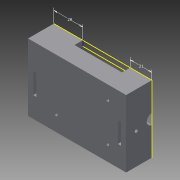
# Autodesk Inventor part: MAINCHAMBER
Saved by Autodesk Inventor 2013 (Build 170138000, 138)
## iProperties
Created: 2013-06-23
Part Number: MAINCHAMBER
Material: Generic
Document SubType Name: Modeling
Designer: Virtual
Density: 1 g/cm^3
Author: Virtual
Autodesk Inventor part; units mm, degrees
ref_plane "YZ Plane" through (0, 0, 0) normal (1, 0, 0) x (0, 1, 0)
ref_plane "XZ Plane" through (0, 0, 0) normal (0, 1, 0) x (-1, 0, 0)
ref_plane "XY Plane" through (0, 0, 0) normal (0, 0, 1) x (1, 0, 0)
sketch "Sketch1" plane through (0, 0, 0) normal (0, 1, 0) x (-1, 0, 0)
  line L0 (0, 0) -> (95, 0)
  line L1 (95, 0) -> (95, 65)
  line L2 (95, 65) -> (0, 65)
  line L3 (0, 65) -> (0, 0)
  dimension "d0" = 95
  dimension "d1" = 65
  constraints: 8 end point, 2 parallel, 1 horizontal, 1 perpendicular
  measures "d0" distance of L2.end L1.end
  measures "d1" distance of L1.end L0.end
extrude "Extrusion1" add sketch "Sketch1" along normal blind 25
sketch "Sketch2" plane through (0, 25, 0) normal (0, 1, 0) x (1, 0, 0)
  line L0 (-5, -5) -> (-90, -5)
  line L1 (-90, -5) -> (-90, -60)
  line L2 (-90, -60) -> (-5, -60)
  line L3 (-5, -60) -> (-5, -5)
  constraints: 8 end point, 2 parallel, 1 horizontal, 1 perpendicular
extrude "Extrusion2" cut sketch "Sketch2" against normal blind 20
sketch "Sketch3" plane through (0, 25, 0) normal (0, 1, 0) x (1, 0, 0)
  line L0 (-5, -60) -> (-90, -60) projected
  line L1 (-95, -65) -> (0, -65) projected
  line L2 (-67, -65) -> (-67, -60)
  line L3 (-21, -60) -> (-21, -65)
  line L4 (-90, -5) -> (-5, -5) projected
  line L5 (0, 0) -> (-95, 0) projected
  line L6 (0, -65) -> (0, 0) projected
  line L7 (-67, -5) -> (-67, 0)
  line L8 (-21, -5) -> (-21, 0)
  line L9 (-67, 0) -> (-21, 0)
  line L10 (-21, -5) -> (-67, -5)
  dimension "d6" = 28
  dimension "d7" = 21
  constraints: 12 end point, 8 point on line, 3 perpendicular, 2 parallel, 1 collinear
  measures "d6" distance of L1.start L2.start
  measures "d7" distance of L1.end L3.end
extrude "Extrusion4" cut sketch "Sketch3" against normal blind 8 contours L3 L1 L2 L0
extrude "Extrusion5" cut sketch "Sketch3" against normal blind 8 contours L8 L4 L7 L5
sketch "Sketch4" plane through (0, 0, 65) normal (1, 0, 0) x (0, 0, -1)
  line L0 (0, 25) -> (65, 25) projected
  circle A0 centre (32.5, 25) radius 5
  dimension "d14" = 10
  constraints: 1 centre point, 1 midpoint
  measures "d14" diameter of A0
extrude "Extrusion6" cut sketch "Sketch4" against normal blind 8
sketch "Sketch5" plane through (0, 5, 0) normal (0, 1, 0) x (1, 0, 0)
  line L0 (-90, -5) -> (-5, -5) projected
  line L1 (-90, -60) -> (-90, -5) projected
  line L2 (-90, -20) -> (-87, -20)
  line L3 (-87, -20) -> (-87, -40)
  line L4 (-87, -40) -> (-90, -40)
  line L5 (-90, -40) -> (-90, -20)
  point P0 (0, 0)
  dimension "d17" = 3
  dimension "d18" = 20
  dimension "d19" = 15
  constraints: 8 end point, 2 parallel, 1 horizontal, 1 perpendicular, 1 point on line
  measures "d17" distance of L3.end L4.end
  measures "d18" distance of L2.end L3.end
  measures "d19" distance between parallel lines of L0 L2
extrude "Extrusion7" cut sketch "Sketch5" against normal blind 8
sketch "Sketch6" plane through (0, 5, 0) normal (0, 1, 0) x (1, 0, 0)
  line L0 (-5, -5) -> (-5, -60) projected
  line L1 (-90, -20) -> (-90, -5) projected
  line L2 (-5, -20) -> (-8, -20)
  line L3 (-8, -20) -> (-8, -40)
  line L4 (-8, -40) -> (-5, -40)
  point P0 (0, 0)
  dimension "d22" = 3
  dimension "d23" = 20
  constraints: 6 end point, 2 perpendicular, 2 point on line, 1 parallel
  measures "d22" distance of L2.start L2.end
  measures "d23" distance of L2.end L3.end
extrude "Extrusion8" cut sketch "Sketch6" against normal blind 8
sketch "Sketch7" plane through (-95, 0, 0) normal (-1, 0, 0) x (0, 0, 1)
  line L0 (0, 0) -> (65, 0) projected
  line L1 (0, 0) -> (0, 25) projected
  circle A0 centre (30, 10) radius 1.625
  dimension "d26" = 3.25
  dimension "d27" = 10
  dimension "d28" = 30
  constraints: 1 centre point
  measures "d26" diameter of A0
  measures "d27" distance from line of A0.centre L0
  measures "d28" distance from line of A0.centre L1
hole "Hole1" at (-95, 10, 30) direction (1, 0, 0) diameter 3.25 end through all
sketch "Sketch8" plane through (0, 5, 0) normal (0, 1, 0) x (1, 0, 0)
  line L0 (-5, -5) -> (-5, -20) projected
  line L1 (-90, -5) -> (-5, -5) projected
  line L2 (-90, -20) -> (-90, -5) projected
  line L3 (-5, -60) -> (-90, -60) projected
  circle A0 centre (-68, -15) radius 1.6
  circle A1 centre (-18, -15) radius 1.6
  circle A2 centre (-18, -52) radius 1.6
  line L4 (-5, -40) -> (-5, -60) projected
  point P0 (0, 0)
  dimension "d36" = 3.2
  dimension "d39" = 3.2
  dimension "d50" = 22
  dimension "d51" = 10
  dimension "d52" = 10
  dimension "d53" = 13
  dimension "d54" = 13
  dimension "d55" = 8
  constraints: 3 centre point
  measures "d36" diameter of A0
  measures "d39" diameter of A1
  measures "d50" distance from line of A0.centre L2
  measures "d51" distance from line of A0.centre L1
  measures "d52" distance from line of L1 A1.centre
  measures "d53" distance from line of L0 A1.centre
  measures "d54" distance from line of L4 A2.centre
  measures "d55" distance from line of L3 A2.centre
hole "Hole2" at (-68, 5, 15) at (-18, 5, 15) at (-18, 5, 52) direction (0, -1, 0) diameter 3.2 end through all
body "Solid1"
